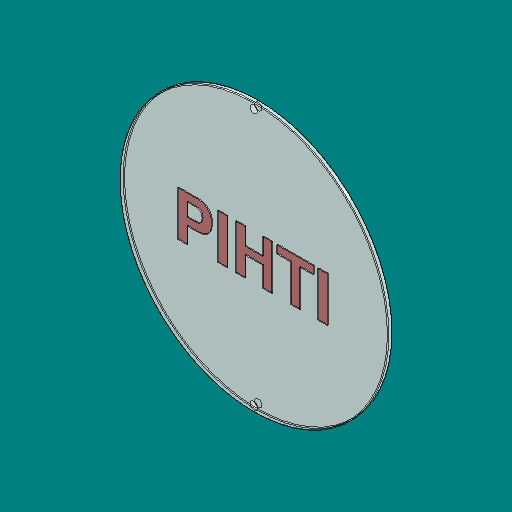
# Autodesk Inventor part: cage-disk-lid
Saved by Autodesk Inventor 2025 (Build 290162000, 162)
## iProperties
Created: 2024-07-04
Part Number: cage-disk-lid
Material: Nylon 6/6
Document SubType Name: Modeling
Designer: kuzmin
Density: 1.13 g/cm^3
Appearance: Clear
Author: kuzmin
Autodesk Inventor part; units mm, degrees
ref_plane "YZ Plane" through (0, 0, 0) normal (1, 0, 0) x (0, 1, 0)
ref_plane "XZ Plane" through (0, 0, 0) normal (0, 1, 0) x (-1, 0, 0)
ref_plane "XY Plane" through (0, 0, 0) normal (0, 0, 1) x (1, 0, 0)
sketch "Sketch1" plane through (0, 0, 0) normal (0, 0, 1) x (1, 0, 0)
  circle A0 centre (0, 0) radius 90
  dimension "d0" = 180
  constraints: 1 centre point, 1 coincident
  measures "d0" diameter of A0
extrude "Extrusion1" add sketch "Sketch1" along normal blind 3
sketch "Sketch2" plane through (0, 0, 3) normal (0, 0, 1) x (1, 0, 0)
  circle A0 centre (0, 0) radius 86 construction
  point P0 (0, 86)
  dimension "d3" = 172
  constraints: 2 vertical alignment, 1 coincident, 2 other
hole "Hole1" at (0, 86, 3) direction (0, 0, -1) diameter 5 end through all
pattern_circular "Circular Pattern1" count 2 over 360 about axis through (0, 0, 0) along (0, 0, 1) of "Hole1"
chamfer "Chamfer1" distance 0.5 angle 45 2 edges at (-90, 0, 3) (-90, 0, 0)
sketch "Sketch3" plane through (0, 0, 3) normal (0, 0, 1) x (1, 0, 0)
  line L0 (-54.241, 15) -> (54.241, 15) construction
  line L1 (54.241, 15) -> (54.241, -15) construction
  line L2 (54.241, -15) -> (-54.241, -15) construction
  line L3 (-54.241, -15) -> (-54.241, 15) construction
  spline S0 degree 2 poles (-28.3154, 5.4931) (-28.3154, 0.1819) (-33.5781, -4.2078) (-38.4528, -4.2078) knots 0 0 0 1 2 2 2
  line L4 (-38.4528, -4.2078) -> (-44.6856, -4.2078)
  line L5 (-44.6856, -4.2078) -> (-44.6856, -15)
  line L6 (-44.6856, -15) -> (-50.9185, -15)
  line L7 (-50.9185, -15) -> (-50.9185, 15)
  line L8 (-50.9185, 15) -> (-38.0648, 15)
  spline S1 degree 2 poles (-38.0648, 15) (-33.6024, 15) (-28.3154, 10.3678) (-28.3154, 5.4931) knots 0 0 0 1 2 2 2
  spline S2 degree 2 poles (-34.5482, 5.4446) (-34.5482, 7.7971) (-36.9249, 9.7858) (-39.0591, 9.7858) knots 0 0 0 1 2 2 2
  line L9 (-39.0591, 9.7858) -> (-44.6856, 9.7858)
  line L10 (-44.6856, 9.7858) -> (-44.6856, 0.958)
  line L11 (-44.6856, 0.958) -> (-39.0591, 0.958)
  spline S3 degree 2 poles (-39.0591, 0.958) (-36.9249, 0.958) (-34.5482, 3.1164) (-34.5482, 5.4446) knots 0 0 0 1 2 2 2
  line L12 (-17.8869, -15) -> (-24.1198, -15)
  line L13 (-24.1198, -15) -> (-24.1198, 15)
  line L14 (-24.1198, 15) -> (-17.8869, 15)
  line L15 (-17.8869, 15) -> (-17.8869, -15)
  line L16 (-12.0907, -15) -> (-12.0907, 15)
  line L17 (-12.0907, 15) -> (-5.8578, 15)
  line L18 (-5.8578, 15) -> (-5.8578, 3.5529)
  line L19 (-5.8578, 3.5529) -> (5.7832, 3.5529)
  line L20 (5.7832, 3.5529) -> (5.7832, 15)
  line L21 (5.7832, 15) -> (12.016, 15)
  line L22 (12.016, 15) -> (12.016, -15)
  line L23 (12.016, -15) -> (5.7832, -15)
  line L24 (5.7832, -15) -> (5.7832, -1.6128)
  line L25 (5.7832, -1.6128) -> (-5.8578, -1.6128)
  line L26 (-5.8578, -1.6128) -> (-5.8578, -15)
  line L27 (-5.8578, -15) -> (-12.0907, -15)
  line L28 (39.8091, 15) -> (39.8091, 9.6888)
  line L29 (39.8091, 9.6888) -> (30.8358, 9.6888)
  line L30 (30.8358, 9.6888) -> (30.8358, -15)
  line L31 (30.8358, -15) -> (24.5302, -15)
  line L32 (24.5302, -15) -> (24.5302, 9.6888)
  line L33 (24.5302, 9.6888) -> (15.5084, 9.6888)
  line L34 (15.5084, 9.6888) -> (15.5084, 15)
  line L35 (15.5084, 15) -> (39.8091, 15)
  line L36 (49.1947, -15) -> (42.9619, -15)
  line L37 (42.9619, -15) -> (42.9619, 15)
  line L38 (42.9619, 15) -> (49.1947, 15)
  line L39 (49.1947, 15) -> (49.1947, -15)
  point P0 (0, 0)
  point P1 (54.241, 0)
  point P2 (0, -15)
  dimension "d17" = 30
  constraints: 2 midpoint, 1 horizontal, 1 horizontal alignment, 1 vertical alignment, 2 other
  measures "d17" distance of L0.end L1.end
emboss "Emboss1" sketch "Sketch3" operation cut depth 0.6 direction (0, 0, -1)
body "Solid1"
